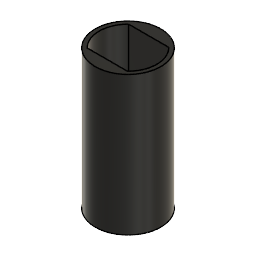
Spacer (Autodesk Fusion 360 design; units mm, degrees)
Autodesk Fusion 360 part; units mm, degrees
sketch "Spacer_Wheel_Ax_Sketch" plane through (0, 0, 0) normal (0, 0, 1) x (1, 0, 0)
  circle A0 centre (0, 0) radius 5
  arc A1 (-3, 3) -> (-3, -3) centre (0, 0) ccw
  line L0 (3, 3) -> (-3, 3)
  arc A2 (3, -3) -> (3, 3) centre (0, 0) ccw
  line L1 (-3, -3) -> (3, -3)
  line L2 (-3.0615, -3.15) -> (3.0615, -3.15)
  arc A3 (3.0615, -3.15) -> (3.0615, 3.15) centre (0, 0) ccw
  line L3 (3.0615, 3.15) -> (-3.0615, 3.15)
  arc A4 (-3.0615, 3.15) -> (-3.0615, -3.15) centre (0, 0) ccw
  dimension "d1" = 0.15
extrude "Extrude1" add sketch "Spacer_Wheel_Ax_Sketch" along normal blind 21.2 contours A0
named bodies: "Spacerr_Body"
